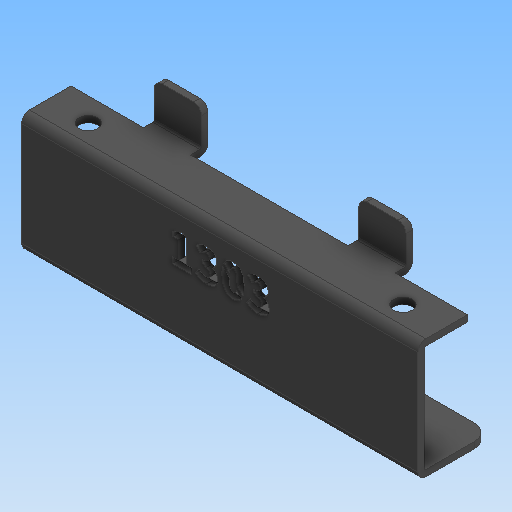
# Autodesk Inventor part: 0 零件
Saved by Autodesk Inventor 2020 (Build 240168000, 168)
## iProperties
Created: 2020-11-03
Part Number: 0 零件
Material: 鋼、碳鋼
Document SubType Name: Sheet Metal
Designer: p2013
Density: 7.85 g/cm^3
Appearance: 一般
Sheet Metal Rule: 預設 mm (_M)
Flat Pattern Width: 8.73053 cm
Flat Pattern Length: 12.6 cm
Flat Pattern Area: 110.005 cm^2
Sheet Metal Width: 87.305 mm
Sheet Metal Length: 126.000 mm
Sheet Metal Area: 11000.469 mm^2
Author: p2013
Autodesk Inventor part; units mm, degrees
ref_plane "YZ Plane" through (0, 0, 0) normal (1, 0, 0) x (0, 1, 0)
ref_plane "XZ Plane" through (0, 0, 0) normal (0, 1, 0) x (-1, 0, 0)
ref_plane "XY Plane" through (0, 0, 0) normal (0, 0, 1) x (1, 0, 0)
sketch "草圖1" plane through (0, 0, 0) normal (0, 0, 1) x (1, 0, 0)
  line L0 (0, -37.8) -> (-54.0641, -37.8) construction
  line L1 (0, -37.8) -> (0, 26.5671) construction
  line L2 (-63, 30.5) -> (63, 30.5)
  line L3 (63, 30.5) -> (63, -37.8)
  line L4 (63, -37.8) -> (-63, -37.8)
  line L5 (-63, -37.8) -> (-63, 30.5)
  line L6 (-63, 16.5) -> (63, 16.5)
  line L7 (-63, -16.5) -> (63, -16.5)
  line L8 (-63, 16.5) -> (63, -16.5) construction
  circle A0 centre (-50, 23) radius 3
  line L9 (0, 4) -> (0, 4) construction
  circle A1 centre (50, 23) radius 3
  line L10 (40, 30.5) -> (25, 30.5)
  line L11 (25, 30.5) -> (25, 46)
  line L12 (27.5, 48.5) -> (37.5, 48.5)
  line L13 (40, 46) -> (40, 30.5)
  line L14 (-40, 30.5) -> (-25, 30.5)
  line L15 (-25, 30.5) -> (-25, 46)
  line L16 (-27.5, 48.5) -> (-37.5, 48.5)
  line L17 (-40, 46) -> (-40, 30.5)
  line L18 (56.1956, 33.5) -> (-56.4376, 33.5)
  arc A2 (40, 46) -> (37.5, 48.5) centre (37.5, 46) ccw
  arc A3 (27.5, 48.5) -> (25, 46) centre (27.5, 46) ccw
  arc A4 (-25, 46) -> (-27.5, 48.5) centre (-27.5, 46) ccw
  arc A5 (-37.5, 48.5) -> (-40, 46) centre (-37.5, 46) ccw
  line L19 (-16.2389, 12) -> (17.2937, 12) construction
  line L20 (17.2937, 12) -> (17.2937, 1.2491) construction
  line L21 (17.2937, 1.2491) -> (-16.2389, 1.2491) construction
  line L22 (-16.2389, 1.2491) -> (-16.2389, 12) construction
  line L23 (-15.1897, 1.8313) -> (-15.1897, 3.7608)
  line L24 (-15.1897, 3.7608) -> (-13.0694, 3.7608)
  line L25 (-13.0694, 3.7608) -> (-13.0694, 9.4395)
  line L26 (-13.0694, 9.4395) -> (-14.9109, 9.4395)
  line L27 (-14.9109, 9.4395) -> (-14.9109, 10.9142)
  spline S0 degree 2 poles (-14.9109, 10.9142) (-13.4509, 11.1856) (-12.4384, 11.8313) knots 0 0 0 1 1 1
  line L28 (-12.4384, 11.8313) -> (-11.558, 11.8313)
  line L29 (-11.558, 11.8313) -> (-10.6849, 10.9582)
  line L30 (-10.6849, 10.9582) -> (-10.6849, 3.7608)
  line L31 (-10.6849, 3.7608) -> (-8.8874, 3.7608)
  line L32 (-8.8874, 3.7608) -> (-8.8874, 1.8313)
  line L33 (-8.8874, 1.8313) -> (-15.1897, 1.8313)
  spline S1 degree 2 poles (-4.324, 1.6405) (-6.547, 1.6405) (-7.7429, 3.0418) knots 0 0 0 1 1 1
  line L34 (-7.7429, 3.0418) -> (-6.6424, 4.5385)
  spline S2 degree 2 poles (-6.6424, 4.5385) (-5.6079, 3.5774) (-4.5661, 3.5774) knots 0 0 0 1 1 1
  spline S3 degree 2 poles (-4.5661, 3.5774) (-3.8544, 3.5774) (-3.4509, 3.8709) knots 0 0 0 1 1 1
  spline S4 degree 2 poles (-3.4509, 3.8709) (-3.0327, 4.1643) (-3.0327, 4.7806) knots 0 0 0 1 1 1
  spline S5 degree 2 poles (-3.0327, 4.7806) (-3.0327, 5.4116) (-4.1039, 6.0866) (-4.4927, 6.0205) knots 0 0 0 1 2 2 2
  line L35 (-4.4927, 6.0205) -> (-5.5859, 6.9596)
  line L36 (-5.5859, 6.9596) -> (-5.5859, 7.774)
  spline S6 degree 2 poles (-5.5859, 7.774) (-4.3606, 7.774) (-3.3408, 8.449) (-3.3408, 9.08) knots 0 0 0 1 2 2 2
  spline S7 degree 2 poles (-3.3408, 9.08) (-3.3408, 10.1365) (-4.4854, 10.1365) knots 0 0 0 1 1 1
  spline S8 degree 2 poles (-4.4854, 10.1365) (-5.3291, 10.1365) (-6.2682, 9.3074) knots 0 0 0 1 1 1
  line L37 (-6.2682, 9.3074) -> (-7.4788, 10.7674)
  spline S9 degree 2 poles (-7.4788, 10.7674) (-6.0114, 12) (-2.7906, 12) (-1.8808, 11.281) knots 0 0 0 1 2 2 2
  spline S10 degree 2 poles (-1.8808, 11.281) (-0.9564, 10.5693) (-0.9564, 9.2487) knots 0 0 0 1 1 1
  spline S11 degree 2 poles (-0.9564, 9.2487) (-0.9564, 7.6933) (-2.5485, 6.9817) knots 0 0 0 1 1 1
  spline S12 degree 2 poles (-2.5485, 6.9817) (-1.6754, 6.7175) (-0.6336, 5.4776) (-0.6336, 4.5532) knots 0 0 0 1 2 2 2
  spline S13 degree 2 poles (-0.6336, 4.5532) (-0.6336, 3.2106) (-1.7047, 2.4182) knots 0 0 0 1 1 1
  spline S14 degree 2 poles (-1.7047, 2.4182) (-2.7686, 1.6405) (-4.324, 1.6405) knots 0 0 0 1 1 1
  spline S15 degree 2 poles (6.7766, 2.9978) (5.8228, 1.6405) (2.5799, 1.6405) (0.6577, 4.3551) (0.6577, 9.3881) (2.5799, 12) (5.8228, 12) (7.7303, 9.3734) (7.7303, 4.3551) (6.7766, 2.9978) knots 0 0 0 1 2 3 4 5 6 7 8 8 8
  spline S16 degree 2 poles (3.2549, 4.2304) (3.5997, 3.4967) (4.803, 3.4967) (5.4779, 4.9714) (5.4779, 8.1775) (5.1111, 9.6963) (4.5902, 10.1805) (3.8125, 10.1805) (3.2769, 9.6963) (2.9101, 8.1775) (2.9101, 4.9714) (3.2549, 4.2304) knots 0 0 0 1 2 3 4 5 6 7 8 9 10 10 10
  spline S17 degree 2 poles (12.0223, 1.6405) (9.7993, 1.6405) (8.6034, 3.0418) knots 0 0 0 1 1 1
  line L38 (8.6034, 3.0418) -> (9.7039, 4.5385)
  spline S18 degree 2 poles (9.7039, 4.5385) (10.7384, 3.5774) (11.7802, 3.5774) knots 0 0 0 1 1 1
  spline S19 degree 2 poles (11.7802, 3.5774) (12.4919, 3.5774) (12.8954, 3.8709) knots 0 0 0 1 1 1
  spline S20 degree 2 poles (12.8954, 3.8709) (13.3136, 4.1643) (13.3136, 4.7806) knots 0 0 0 1 1 1
  spline S21 degree 2 poles (13.3136, 4.7806) (13.3136, 5.4116) (12.2424, 6.0866) (11.8536, 6.0205) knots 0 0 0 1 2 2 2
  line L39 (11.8536, 6.0205) -> (10.7604, 6.9596)
  line L40 (10.7604, 6.9596) -> (10.7604, 7.774)
  spline S22 degree 2 poles (10.7604, 7.774) (11.9856, 7.774) (13.0055, 8.449) (13.0055, 9.08) knots 0 0 0 1 2 2 2
  spline S23 degree 2 poles (13.0055, 9.08) (13.0055, 10.1365) (11.8609, 10.1365) knots 0 0 0 1 1 1
  spline S24 degree 2 poles (11.8609, 10.1365) (11.0172, 10.1365) (10.0781, 9.3074) knots 0 0 0 1 1 1
  line L41 (10.0781, 9.3074) -> (8.8675, 10.7674)
  spline S25 degree 2 poles (8.8675, 10.7674) (10.3349, 12) (13.5557, 12) (14.4655, 11.281) knots 0 0 0 1 2 2 2
  spline S26 degree 2 poles (14.4655, 11.281) (15.3899, 10.5693) (15.3899, 9.2487) knots 0 0 0 1 1 1
  spline S27 degree 2 poles (15.3899, 9.2487) (15.3899, 7.6933) (13.7978, 6.9817) knots 0 0 0 1 1 1
  spline S28 degree 2 poles (13.7978, 6.9817) (14.6709, 6.7175) (15.7127, 5.4776) (15.7127, 4.5532) knots 0 0 0 1 2 2 2
  spline S29 degree 2 poles (15.7127, 4.5532) (15.7127, 3.2106) (14.6416, 2.4182) knots 0 0 0 1 1 1
  spline S30 degree 2 poles (14.6416, 2.4182) (13.5777, 1.6405) (12.0223, 1.6405) knots 0 0 0 1 1 1
  point P0 (0, 0)
  point P1 (0, 0)
  point P2 (25, 48.5)
  point P3 (40, 48.5)
  point P4 (-25, 48.5)
  point P5 (-40, 48.5)
  point P6 (25, 30.5)
  point P7 (-40, 30.5)
  point P8 (-25, 30.5)
  dimension "d0" = 126
  dimension "d1" = 21.3
  dimension "d2" = 33
  dimension "d3" = 14
  dimension "d11" = 6
  dimension "d12" = 7.5
  dimension "d15" = 0
  dimension "d18" = 100
  dimension "d25" = 15
  dimension "d26" = 80
  dimension "d28" = 3
  dimension "d31" = 2.5
  dimension "d32" = 15
  dimension "d36" = 4.5
  constraints: 38 end point, 13 point on line, 8 point on circle, 8 tangent, 6 centre point, 5 horizontal, 5 symmetric about line, 4 parallel, 4 perpendicular, 3 equal radius, 2 midpoint, 2 vertical, 1 coincident, 4 other
  measures "d0" distance between parallel lines of L3 L5
  measures "d1" distance between parallel lines of L7 L4
  measures "d2" distance between parallel lines of L6 L7
  measures "d3" distance between parallel lines of L6 L2
  measures "d11" diameter of A0
  measures "d12" distance from line of A0.centre L2
  measures "d15" distance of L9.end L9.start
  measures "d18" distance of A1.centre A0.centre
  measures "d25" distance between parallel lines of L11 L13
  measures "d26" distance between parallel lines of L17 L13
  measures "d28" distance between parallel lines of L2 L18
  measures "d31" radius of A2
  measures "d32" distance between parallel lines of L18 L12
  measures "d36" distance between parallel lines of L6 L19
extrude "擠出1" add sketch "草圖1" along normal blind 2 contours L2 L3 L6 L5 | L17 L18 L15 L2 | L6 L3 L7 L5 | L17 A5 L16 A4 L15 L18 | L7 L3 L4 L5 | L11 L18 L13 L2 | L11 A3 L12 A2 L13 L18 | L23 L24 L25 L26 L27 S0 L28 L29 L30 L31 L32 L33 | S1 L34 S2 S3 S4 S5 L35 L36 S6 S7 S8 L37 S9 S10 S11 S12 S13 S14 | S15 | S16 | S17 L38 S18 S19 S20 S21 L39 L40 S22 S23 S24 L41 S25 S26 S27 S28 S29 S30
extrude "擠出3" cut sketch "草圖1" along normal up to surface (2 mm away) contours L23 L24 L25 L26 L27 S0 L28 L29 L30 L31 L32 L33 | S1 L34 S2 S3 S4 S5 L35 L36 S6 S7 S8 L37 S9 S10 S11 S12 S13 S14 | S15 | S17 L38 S18 S19 S20 S21 L39 L40 S22 S23 S24 L41 S25 S26 S27 S28 S29 S30
sketch "草圖4" plane through (0, 0, 2) normal (0, 0, 1) x (1, 0, 0)
  spline S0 degree 2 poles (6.7766, 2.9978) (5.8228, 1.6405) (2.5799, 1.6405) (0.6577, 4.3551) (0.6577, 9.3881) (2.5799, 12) (5.8228, 12) (7.7303, 9.3734) (7.7303, 4.3551) (6.7766, 2.9978) knots 0 0 0 0.125 0.25 0.375 0.5 0.625 0.75 0.875 1 1 1 projected
  spline S1 degree 2 poles (3.2549, 4.2304) (3.5997, 3.4967) (4.803, 3.4967) (5.4779, 4.9714) (5.4779, 8.1775) (5.1111, 9.6963) (4.5902, 10.1805) (3.8125, 10.1805) (3.2769, 9.6963) (2.9101, 8.1775) (2.9101, 4.9714) (3.2549, 4.2304) knots 0 0 0 0.1 0.2 0.3 0.4 0.5 0.6 0.7 0.8 0.9 1 1 1 projected
  line L0 (0, 10.0218) -> (7.4981, 2.5237)
  line L1 (0.7071, 10.7289) -> (8.2052, 3.2308)
  line L2 (0, 10.0218) -> (0.7071, 10.7289)
  line L3 (7.4981, 2.5237) -> (8.2052, 3.2308)
  line L4 (0, 65.76) -> (0, -55.06) projected
  point P0 (0, 0)
  point P1 (7.3325, 4.1035)
  point P2 (5.4646, 5.9714)
  point P3 (5.3038, 4.718)
  point P4 (6.8757, 3.1461)
  point P5 (3.0035, 8.4325)
  point P6 (1.2861, 10.1499)
  point P7 (0.9057, 9.116)
  point P8 (2.9156, 7.1062)
  dimension "d45" = 45
  dimension "d46" = 1
  dimension "d47" = 7.4981
  dimension "d48" = 10.0218
  constraints: 8 end point, 2 parallel, 1 perpendicular, 1 point on line, 1 vertical alignment, 2 other
  measures "d45" angle of L4 L1
  measures "d46" distance between parallel lines of L0 L1
  measures "d47" horizontal distance of L1.start L1.end
  measures "d48" distance of point (0, 0) L0.start
extrude "擠出4" add sketch "草圖4" against normal up to surface (2 mm away) contours S0 L1 S1 L0 | L0 S1 L1 S0
bend part "折彎零件3" radius 2.5 angle 90 line through (56.1956, 33.5, 0) along (-1, 0, 0) centre toward (0, 0, 1) moving side (0, 1, 0) both sides no
bend part "折彎零件1" radius 0.5 angle 90 line through (-63, 16.5, 0) along (1, 0, 0) centre toward (0, 0, -1) moving side (0, 1, 0) both sides no
bend part "折彎零件2" radius 0.5 angle 90 line through (-63, -16.5, 0) along (1, 0, 0) centre toward (0, 0, -1) moving side (0, -1, 0) both sides no
fillet "圓角1" radius 5 2 edges at (63, -18, -21.0146) (-63, -18, -21.0146)
